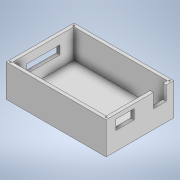
# Autodesk Inventor part: remoteswitchbox
Saved by Autodesk Inventor 2021 (Build 250183000, 183)
## iProperties
Created: 2021-10-23
Part Number: remoteswitchbox
Material: Generic
Document SubType Name: Modeling
Designer: eddys
Density: 1 g/cm^3
Appearance: Default
Author: eddys
Autodesk Inventor part; units mm, degrees
ref_plane "YZ Plane" through (0, 0, 0) normal (1, 0, 0) x (0, 1, 0)
ref_plane "XZ Plane" through (0, 0, 0) normal (0, 1, 0) x (-1, 0, 0)
ref_plane "XY Plane" through (0, 0, 0) normal (0, 0, 1) x (1, 0, 0)
sketch "Sketch1" plane through (0, 0, 0) normal (0, 1, 0) x (-1, 0, 0)
  line L0 (46.5, 31.5) -> (-46.5, 31.5)
  line L1 (-46.5, 31.5) -> (-46.5, -31.5)
  line L2 (-46.5, -31.5) -> (46.5, -31.5)
  line L3 (46.5, -31.5) -> (46.5, 31.5)
  line L4 (46.5, 31.5) -> (-46.5, -31.5) construction
  line L5 (-46.5, 31.5) -> (46.5, -31.5) construction
  point P0 (0, 0)
  dimension "d0" = 63
  dimension "d1" = 93
  constraints: 12 end point, 2 midpoint, 2 parallel, 1 horizontal, 1 perpendicular
  measures "d0" distance of L2.end L0.start
  measures "d1" distance of L1.end L2.end
extrude "Extrusion1" add sketch "Sketch1" along normal blind 3
sketch "Sketch2" plane through (0, 3, 0) normal (0, 1, 0) x (1, 0, 0)
  line L0 (-43.5, -28.5) -> (43.5, -28.5)
  line L1 (43.5, -28.5) -> (43.5, 28.5)
  line L2 (43.5, 28.5) -> (-43.5, 28.5)
  line L3 (-43.5, 28.5) -> (-43.5, -28.5)
  line L4 (-43.5, -28.5) -> (43.5, 28.5) construction
  line L5 (43.5, -28.5) -> (-43.5, 28.5) construction
  line L6 (46.5, -31.5) -> (46.5, 31.5) projected
  line L7 (-46.5, -31.5) -> (46.5, -31.5)
  line L8 (46.5, -31.5) -> (46.5, 31.5)
  line L9 (46.5, 31.5) -> (-46.5, 31.5)
  line L10 (-46.5, 31.5) -> (-46.5, -31.5)
  line L11 (-46.5, -31.5) -> (46.5, 31.5) construction
  line L12 (46.5, -31.5) -> (-46.5, 31.5) construction
  point P0 (0, 0)
  point P1 (46.5, -31.5)
  dimension "d4" = 57
  dimension "d5" = 87
  constraints: 24 end point, 4 midpoint, 4 parallel, 2 horizontal, 2 perpendicular
  measures "d4" distance of L2.end L0.start
  measures "d5" distance of L1.end L2.end
extrude "Extrusion2" add sketch "Sketch2" along normal blind 27
sketch "Sketch3" plane through (0, 30, 0) normal (0, 1, 0) x (1, 0, 0)
  circle A0 centre (-44.5, 29.5) radius 0.75
  line L0 (46.5, 31.5) -> (-46.5, 31.5) projected
  line L1 (-46.5, 31.5) -> (-46.5, -31.5) projected
  circle A1 centre (-44.5, -29.5) radius 0.75
  line L2 (-46.5, -31.5) -> (46.5, -31.5) projected
  circle A2 centre (44.5, -29.5) radius 0.75
  line L3 (46.5, -31.5) -> (46.5, 31.5) projected
  circle A3 centre (44.5, 29.5) radius 0.75
  point P0 (0, 0)
  dimension "d8" = 2
  dimension "d9" = 2
  dimension "d10" = 1.5
  dimension "d11" = 2
  dimension "d12" = 2
  dimension "d13" = 1.5
  dimension "d14" = 2
  dimension "d15" = 2
  dimension "d16" = 1.5
  dimension "d17" = 2
  dimension "d18" = 2
  dimension "d19" = 1.5
  constraints: 4 centre point
  measures "d8" distance from line of L0 A0.centre
  measures "d9" distance from line of L1 A0.centre
  measures "d10" diameter of A0
  measures "d11" distance from line of L1 A1.centre
  measures "d12" distance from line of L2 A1.centre
  measures "d13" diameter of A1
  measures "d14" distance from line of L3 A2.centre
  measures "d15" distance from line of L2 A2.centre
  measures "d16" diameter of A2
  measures "d17" distance from line of L0 A3.centre
  measures "d18" distance from line of L3 A3.centre
  measures "d19" diameter of A3
extrude "Extrusion3" cut sketch "Sketch3" against normal blind 5 contours A0 | A1 | A2 | A3
sketch "Sketch5" plane through (-46.5, 0, -31.5) normal (-1, 0, 0) x (0, 0, 1)
  line L0 (16, 14) -> (47, 14)
  line L1 (47, 14) -> (47, 22)
  line L2 (47, 22) -> (16, 22)
  line L3 (16, 22) -> (16, 14)
  line L4 (0, 0) -> (63, 0) projected
  line L5 (0, 0) -> (0, 30) projected
  point P0 (31.5, 0)
  dimension "d23" = 14
  dimension "d24" = 8
  dimension "d25" = 31
  dimension "d26" = 16
  constraints: 8 end point, 2 parallel, 1 horizontal, 1 perpendicular
  measures "d23" distance between parallel lines of L4 L0
  measures "d24" distance of L0.end L1.end
  measures "d25" distance of L1.end L2.end
  measures "d26" distance between parallel lines of L5 L3
extrude "Extrusion4" cut sketch "Sketch5" against normal blind 3
sketch "Sketch6" plane through (46.5, 0, 31.5) normal (1, 0, 0) x (0, 0, -1)
  line L0 (44, 30) -> (56, 30)
  line L1 (56, 30) -> (56, 17)
  line L2 (56, 17) -> (44, 17)
  line L3 (44, 17) -> (44, 30)
  line L4 (0, 0) -> (63, 0) projected
  line L5 (63, 0) -> (63, 30) projected
  line L6 (9, 26) -> (26, 26)
  line L7 (26, 26) -> (26, 17)
  line L8 (26, 17) -> (9, 17)
  line L9 (9, 17) -> (9, 26)
  line L10 (0, 0) -> (0, 30) projected
  point P0 (31.5, 0)
  dimension "d30" = 17
  dimension "d31" = 13
  dimension "d32" = 12
  dimension "d33" = 7
  dimension "d34" = 9
  dimension "d35" = 17
  dimension "d36" = 17
  dimension "d37" = 9
  constraints: 16 end point, 4 parallel, 2 horizontal, 2 perpendicular
  measures "d30" distance between parallel lines of L4 L2
  measures "d31" distance of L0.end L1.end
  measures "d32" distance between parallel lines of L1 L3
  measures "d33" distance between parallel lines of L5 L1
  measures "d34" distance between parallel lines of L10 L9
  measures "d35" distance of L6.start L6.end
  measures "d36" distance between parallel lines of L4 L8
  measures "d37" distance of L6.end L7.end
extrude "Extrusion5" cut sketch "Sketch6" against normal blind 3
body "Solid1"
